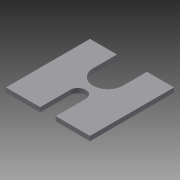
# Autodesk Inventor part: torchArm
Saved by Autodesk Inventor 2013 (Build 170138000, 138)
## iProperties
Created: 2012-12-09
Part Number: torchArm
Material: Generic
Document SubType Name: Modeling
Designer: Istvan
Density: 1 g/cm^3
Mass: 29.3071 g
Surface Area: 145.469 cm^2
Volume: 29.3071 cm^3
Author: Istvan
Autodesk Inventor part; units mm, degrees
ref_plane "YZ Plane" through (0, 0, 0) normal (1, 0, 0) x (0, 1, 0)
ref_plane "XZ Plane" through (0, 0, 0) normal (0, 1, 0) x (-1, 0, 0)
ref_plane "XY Plane" through (0, 0, 0) normal (0, 0, 1) x (1, 0, 0)
sketch "Sketch1" plane through (0, 0, 0) normal (0, 1, 0) x (-1, 0, 0)
  line L0 (0, 0) -> (28.575, 0)
  line L1 (44.45, 41.275) -> (44.45, 58.039)
  line L2 (26.289, 88.9) -> (0, 88.9)
  line L3 (0, 88.9) -> (0, 0)
  line L4 (26.289, 88.9) -> (16.9101, 88.9)
  line L5 (26.289, 76.2) -> (26.289, 88.9)
  arc A0 (26.289, 76.2) -> (44.45, 58.039) centre (44.45, 76.2) ccw
  line L6 (14.2875, 0) -> (28.575, 0)
  line L7 (28.575, 0) -> (28.575, 25.4)
  arc A1 (44.45, 41.275) -> (28.575, 25.4) centre (44.45, 25.4) ccw
  dimension "d2" = 18.161
  dimension "d8" = 12.7
  dimension "d9" = 88.9
  dimension "d11" = 44.45
  dimension "d14" = 25.4
  dimension "d15" = 15.875
  constraints: 16 end point, 5 horizontal, 4 point on circle, 2 centre point, 2 coincident, 2 parallel, 2 perpendicular, 2 tangent, 1 line through centre, 1 midpoint, 1 point on line, 1 vertical, 5 other
  measures "d2" radius of A0
  measures "d8" distance of L2.start L5.start
  measures "d9" distance of L2.end L0.start
  measures "d11" distance between parallel lines of L3 L1
  measures "d14" distance of L0.end L7.end
  measures "d15" radius of A1
extrude "Extrusion1" add sketch "Sketch1" along normal blind 4.7625
mirror "Mirror1" about plane through (-44.45, 0, 41.275) normal (-1, 0, 0)
body "Solid1"
